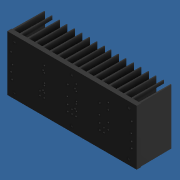
# Autodesk Inventor part: J002135
Saved by Autodesk Inventor 2012 SP2 (Build 160219200, 219)
## iProperties
Created: 2013-05-09
Part Number: J002135
Material: ALUMINUM, 6061-T651
Document SubType Name: Modeling
Designer: RICK
Mass: 816.805 g
Surface Area: 2050.09 cm^2
Volume: 302.52 cm^3
Density: 2.7 g/cm^3
Vendor: HHMI: JFRC - ID&F
Description: MODIFIED HEATSINK
Project: P-119101
ALTERED ITEM DESCRIPTION: HEATSINK
ALTERED ITEM PART NUMBER: 62725
ALTERED ITEM VENDOR: AAVID THERMALLOY
DESIGN DEPARTMENT: HHMI: JFRC - ID&F
SPECIAL FINISH: NONE
SURFACE ROUGHNESS: 125 Ra
Revision Number: 0
Autodesk Inventor part; units mm, degrees
ref_plane "YZ Plane" through (0, 0, 0) normal (1, 0, 0) x (0, 1, 0)
sketch "Sketch1" plane through (0, 0, 0) normal (0, 0, 1) x (1, 0, 0)
  line L0 (-104.14, 88.9) -> (104.14, 88.9)
  line L1 (104.14, 88.9) -> (104.14, 0)
  line L2 (104.14, 0) -> (-104.14, 0)
  line L3 (-104.14, 0) -> (-104.14, 88.9)
  point P0 (0, 0)
  dimension "d1" = 208.28
  dimension "d2" = 88.9
  dimension "d3" = 104.14
  constraints: 8 end point, 2 horizontal, 2 vertical, 1 midpoint
  measures "d1" distance of L0.start L0.end
  measures "d2" distance of L2.end L0.start
  measures "d3" distance from line of L3 point (0, 0)
extrude "Extrusion1" add sketch "Sketch1" against normal blind 7.112
hole "Hole3" at (0, 8.89, 0) direction (0, 0, -1) diameter 3.7973 depth 7.239 tip angle 118
hole "Hole4" at (0, 80.01, 0) direction (0, 0, -1) diameter 3.7973 depth 7.239 tip angle 118
hole "Hole5" at (-91.948, 8.89, 0) direction (0, 0, -1) diameter 3.7973 depth 7.239 tip angle 118
hole "Hole6" at (-91.948, 80.01, 0) direction (0, 0, -1) diameter 3.7973 depth 7.239 tip angle 118
hole "Hole7" at (91.948, 8.89, 0) direction (0, 0, -1) diameter 3.7973 depth 7.239 tip angle 118
hole "Hole8" at (91.948, 80.01, 0) direction (0, 0, -1) diameter 3.7973 depth 7.239 tip angle 118
hole "Hole9" at (-95.504, 46.609, 0) direction (0, 0, -1) diameter 2.159 depth 7.62 tip angle 118
hole "Hole10" at (-44.069, 46.609, 0) direction (0, 0, -1) diameter 2.159 depth 7.62 tip angle 118
hole "Hole11" at (-51.435, 32.258, 0) direction (0, 0, -1) diameter 2.159 depth 7.62 tip angle 118
hole "Hole12" at (-7.366, 46.609, 0) direction (0, 0, -1) diameter 2.159 depth 7.62 tip angle 118
hole "Hole13" at (7.366, 46.609, 0) direction (0, 0, -1) diameter 2.159 depth 7.62 tip angle 118
hole "Hole14" at (0, 32.258, 0) direction (0, 0, -1) diameter 2.159 depth 7.62 tip angle 118
hole "Hole15" at (44.069, 46.609, 0) direction (0, 0, -1) diameter 2.159 depth 7.62 tip angle 118
hole "Hole16" at (51.435, 32.258, 0) direction (0, 0, -1) diameter 2.159 depth 7.62 tip angle 118
hole "Hole17" at (95.504, 46.609, 0) direction (0, 0, -1) diameter 2.159 depth 7.62 tip angle 118
hole "Hole18" at (-97.79, 35.56, 0) direction (0, 0, -1) diameter 2.6416 depth 7.62 tip angle 118 thread size "6-32 UNC" class "2B" standard "ANSI Unified Screw Threads"
hole "Hole19" at (-44.45, 43.18, 0) direction (0, 0, -1) diameter 2.6416 depth 7.62 tip angle 118 thread size "6-32 UNC" class "2B" standard "ANSI Unified Screw Threads"
hole "Hole20" at (-46.482, 35.56, 0) direction (0, 0, -1) diameter 2.6416 depth 7.62 tip angle 118 thread size "6-32 UNC" class "2B" standard "ANSI Unified Screw Threads"
hole "Hole21" at (-44.45, 33.02, 0) direction (0, 0, -1) diameter 2.6416 depth 7.62 tip angle 118 thread size "6-32 UNC" class "2B" standard "ANSI Unified Screw Threads"
hole "Hole22" at (-6.858, 35.56, 0) direction (0, 0, -1) diameter 2.6416 depth 7.62 tip angle 118 thread size "6-32 UNC" class "2B" standard "ANSI Unified Screw Threads"
hole "Hole23" at (6.985, 43.18, 0) direction (0, 0, -1) diameter 2.6416 depth 7.62 tip angle 118 thread size "6-32 UNC" class "2B" standard "ANSI Unified Screw Threads"
hole "Hole24" at (5.08, 35.56, 0) direction (0, 0, -1) diameter 2.6416 depth 7.62 tip angle 118 thread size "6-32 UNC" class "2B" standard "ANSI Unified Screw Threads"
hole "Hole25" at (6.985, 33.02, 0) direction (0, 0, -1) diameter 2.6416 depth 7.62 tip angle 118 thread size "6-32 UNC" class "2B" standard "ANSI Unified Screw Threads"
hole "Hole26" at (44.577, 35.56, 0) direction (0, 0, -1) diameter 2.6416 depth 7.62 tip angle 118 thread size "6-32 UNC" class "2B" standard "ANSI Unified Screw Threads"
hole "Hole27" at (58.42, 43.18, 0) direction (0, 0, -1) diameter 2.6416 depth 7.62 tip angle 118 thread size "6-32 UNC" class "2B" standard "ANSI Unified Screw Threads"
hole "Hole28" at (58.42, 33.02, 0) direction (0, 0, -1) diameter 2.6416 depth 7.62 tip angle 118 thread size "6-32 UNC" class "2B" standard "ANSI Unified Screw Threads"
hole "Hole29" at (96.012, 35.56, 0) direction (0, 0, -1) diameter 2.6416 depth 7.62 tip angle 118 thread size "6-32 UNC" class "2B" standard "ANSI Unified Screw Threads"
sketch "Sketch2" plane through (-104.14, 88.9, 0) normal (0, 1, 0) x (1, 0, 0)
  line L0 (98.1075, 57.1342) -> (97.4963, 7.112)
  line L1 (97.4963, 7.112) -> (100.2933, 7.112)
  line L2 (100.2933, 7.112) -> (99.6822, 57.1342)
  line L3 (208.28, 7.112) -> (0, 7.112) projected
  arc A0 (99.6822, 57.1342) -> (98.1075, 57.1342) centre (98.8948, 57.1246) ccw
  line L4 (0, 0) -> (208.28, 0) projected
  point P0 (104.14, 0)
  dimension "d267" = 6.0325
  dimension "d268" = 1.5748
  dimension "d270" = 57.912
  dimension "d276" = 89.3
  dimension "d278" = 89.3
  dimension "d279" = 2.797
  constraints: 6 end point, 2 point on circle, 2 tangent, 1 centre point, 1 collinear
  measures "d267" horizontal distance of point (104.14, 0) L0.start
  measures "d268" diameter of A0
  measures "d276" angle of L1 L2
  measures "d278" angle of L0 L1
  measures "d279" distance of L1.end L0.end
extrude "Extrusion2" add sketch "Sketch2" against normal blind 88.9
ref_plane "Work Plane2" through (0, 0, 0) normal (-1, 0, 0) x (0, 0, 1)
pattern_linear "Rectangular Pattern1" count 9 spacing 12.065 along (-1, 0, 0) of "Extrusion2"
mirror "Mirror1" about plane through (0, 0, 0) normal (-1, 0, 0) of "Extrusion2", "Rectangular Pattern1"
ref_plane "Work Plane3" through (-104.14, 44.45, 0) normal (0, -1, 0) x (1, 0, 0)
sketch "Sketch4" plane through (0, 0, -7.112) normal (0, 0, -1) x (-1, 0, 0)
  circle A0 centre (-91.948, 8.89) radius 4.7625
  arc A1 (-91.0987, 10.5881) -> (-91.0987, 7.1919) centre (-91.948, 8.89) ccw projected
  point P0 (0, 0)
  dimension "d289" = 9.525
  constraints: 1 centre point, 1 concentric
  measures "d289" diameter of A0
extrude "Extrusion4" cut sketch "Sketch4" along normal blind 63.5
mirror "Mirror4" about plane through (0, 0, 0) normal (-1, 0, 0) of "Extrusion4"
mirror "Mirror5" about plane through (-104.14, 44.45, 0) normal (0, -1, 0) of "Extrusion4", "Mirror4"
hole "Hole30" at (-96.139, 25.7556, 0) direction (0, 0, -1) diameter 2.6416 depth 7.62 tip angle 118 thread size "6-32 UNC" class "2B" standard "ANSI Unified Screw Threads"
hole "Hole31" at (-51.435, 25.7556, 0) direction (0, 0, -1) diameter 2.6416 depth 7.62 tip angle 118 thread size "6-32 UNC" class "2B" standard "ANSI Unified Screw Threads"
hole "Hole32" at (-44.577, 25.7556, 0) direction (0, 0, -1) diameter 2.6416 depth 7.62 tip angle 118 thread size "6-32 UNC" class "2B" standard "ANSI Unified Screw Threads"
hole "Hole33" at (-6.731, 25.7556, 0) direction (0, 0, -1) diameter 2.6416 depth 7.62 tip angle 118 thread size "6-32 UNC" class "2B" standard "ANSI Unified Screw Threads"
hole "Hole34" at (0.127, 25.7556, 0) direction (0, 0, -1) diameter 2.6416 depth 7.62 tip angle 118 thread size "6-32 UNC" class "2B" standard "ANSI Unified Screw Threads"
hole "Hole35" at (6.731, 25.7556, 0) direction (0, 0, -1) diameter 2.6416 depth 7.62 tip angle 118 thread size "6-32 UNC" class "2B" standard "ANSI Unified Screw Threads"
hole "Hole36" at (44.831, 25.7556, 0) direction (0, 0, -1) diameter 2.6416 depth 7.62 tip angle 118 thread size "6-32 UNC" class "2B" standard "ANSI Unified Screw Threads"
hole "Hole37" at (51.435, 25.7556, 0) direction (0, 0, -1) diameter 2.6416 depth 7.62 tip angle 118 thread size "6-32 UNC" class "2B" standard "ANSI Unified Screw Threads"
hole "Hole38" at (96.139, 25.7556, 0) direction (0, 0, -1) diameter 2.6416 depth 7.62 tip angle 118 thread size "6-32 UNC" class "2B" standard "ANSI Unified Screw Threads"
hole "Hole39" at (-44.45, 60.833, 0) direction (0, 0, -1) diameter 2.6416 depth 7.62 tip angle 118 thread size "6-32 UNC" class "2B" standard "ANSI Unified Screw Threads"
hole "Hole40" at (6.985, 60.833, 0) direction (0, 0, -1) diameter 2.6416 depth 7.62 tip angle 118 thread size "6-32 UNC" class "2B" standard "ANSI Unified Screw Threads"
hole "Hole41" at (58.42, 60.833, 0) direction (0, 0, -1) diameter 2.6416 depth 7.62 tip angle 118 thread size "6-32 UNC" class "2B" standard "ANSI Unified Screw Threads"
hole "Hole42" at (-44.45, 70.993, 0) direction (0, 0, -1) diameter 2.6416 depth 7.62 tip angle 118 thread size "6-32 UNC" class "2B" standard "ANSI Unified Screw Threads"
hole "Hole43" at (6.985, 70.993, 0) direction (0, 0, -1) diameter 2.6416 depth 7.62 tip angle 118 thread size "6-32 UNC" class "2B" standard "ANSI Unified Screw Threads"
hole "Hole45" at (-97.917, 63.5, 0) direction (0, 0, -1) diameter 2.6416 depth 7.62 tip angle 118 thread size "6-32 UNC" class "2B" standard "ANSI Unified Screw Threads"
hole "Hole44" at (58.42, 70.993, 0) direction (0, 0, -1) diameter 2.6416 depth 7.62 tip angle 118 thread size "6-32 UNC" class "2B" standard "ANSI Unified Screw Threads"
hole "Hole46" at (-6.731, 63.5, 0) direction (0, 0, -1) diameter 2.6416 depth 7.62 tip angle 118 thread size "6-32 UNC" class "2B" standard "ANSI Unified Screw Threads"
hole "Hole47" at (-46.355, 63.5, 0) direction (0, 0, -1) diameter 2.6416 depth 7.62 tip angle 118 thread size "6-32 UNC" class "2B" standard "ANSI Unified Screw Threads"
hole "Hole48" at (44.831, 63.5, 0) direction (0, 0, -1) diameter 2.6416 depth 7.62 tip angle 118 thread size "6-32 UNC" class "2B" standard "ANSI Unified Screw Threads"
hole "Hole49" at (4.953, 63.5, 0) direction (0, 0, -1) diameter 2.6416 depth 7.62 tip angle 118 thread size "6-32 UNC" class "2B" standard "ANSI Unified Screw Threads"
hole "Hole50" at (96.139, 63.5, 0) direction (0, 0, -1) diameter 2.6416 depth 200.279 tip angle 118 thread size "6-32 UNC" class "2B" standard "ANSI Unified Screw Threads"
equation "\"d3\" = 0.5 * d1"
equation "\"d276\" = d278"
body "Solid1"
